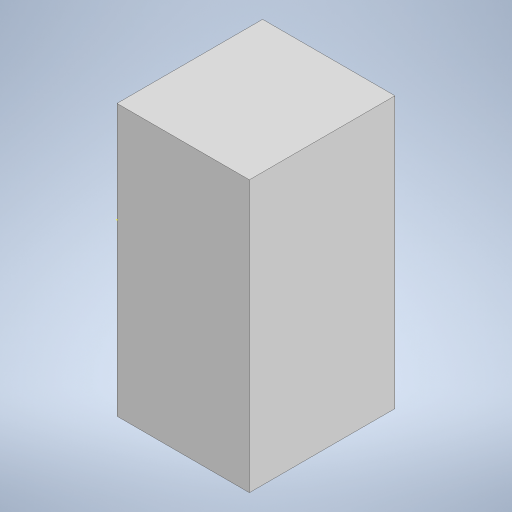
# Autodesk Inventor part: semaforoEsboço
Saved by Autodesk Inventor 2024 (Build 280153020, 153B)
## iProperties
Created: 2023-11-16
Part Number: semaforoEsboço
Material: Genérico
Document SubType Name: Modeling
Designer: a2625288
Density: 1 g/cm^3
Appearance: Padrão
Author: a2625288
Autodesk Inventor part; units mm, degrees
ref_plane "YZ Plane" through (0, 0, 0) normal (1, 0, 0) x (0, 1, 0)
ref_plane "XZ Plane" through (0, 0, 0) normal (0, 1, 0) x (-1, 0, 0)
ref_plane "XY Plane" through (0, 0, 0) normal (0, 0, 1) x (1, 0, 0)
sketch "Esboço1" plane through (0, 0, 0) normal (1, 0, 0) x (0, 1, 0)
  line L0 (10.9206, 18.8054) -> (-21.8794, 18.8054)
  line L1 (-21.8794, 18.8054) -> (-21.8794, 2.1054)
  line L2 (-21.8794, 2.1054) -> (10.9206, 2.1054)
  line L3 (10.9206, 2.1054) -> (10.9206, 18.8054)
  circle A0 centre (4.3506, 9.8054) radius 3.25
  circle A1 centre (4.3506, 9.8054) radius 3.8294
  circle A2 centre (-5.1194, 9.8054) radius 3.25
  circle A3 centre (-5.1194, 9.8054) radius 3.8763
  circle A4 centre (-14.5894, 9.8054) radius 3.25
  circle A5 centre (-14.5894, 9.8054) radius 3.9245
  point P0 (0, 0)
  point P1 (-5.4794, 18.8054)
  dimension "d0" = 32.8
  dimension "d1" = 16.7
  dimension "d2" = 32.8
  dimension "d7" = 6.5
  dimension "d8" = 6.5
  dimension "d9" = 6.5
  dimension "d22" = 9
  dimension "d23" = 9
  dimension "d24" = 9
  constraints: 8 end point, 6 centre point, 3 coincident, 2 perpendicular, 1 horizontal, 1 midpoint
  measures "d0" distance of L0.start L0.end
  measures "d1" distance of L0.end L1.end
  measures "d2" distance of L1.end L2.end
  measures "d7" diameter of A0
  measures "d8" diameter of A2
  measures "d9" diameter of A4
  measures "d22" distance from line of L0 A0.centre
  measures "d23" vertical distance of point (-5.479, 18.805) A2.centre
  measures "d24" distance from line of L0 A4.centre
extrude "Extrusão1" add sketch "Esboço1" along normal blind 3 contours L3 L2 L1 L0
sketch "Esboço2" plane through (0, -21.8794, 18.8054) normal (0, 0, 1) x (1, 0, 0)
  line L0 (3, 0) -> (3, 32.8) projected
  line L1 (0, 32.8) -> (3, 32.8) projected
  line L2 (3, 32.8) -> (15, 32.8)
  line L3 (15, 32.8) -> (15, 0)
  line L4 (15, 0) -> (3, 0)
  point P0 (0, 21.8794)
  dimension "d13" = 12
  constraints: 6 end point, 2 perpendicular, 1 horizontal
  measures "d13" distance of L0.end L2.end
extrude "Extrusão2" add sketch "Esboço2" against normal blind 2
sketch "Esboço3" plane through (0, -21.8794, 16.8054) normal (0, 0, -1) x (-1, 0, 0)
  line L0 (0, 32.8) -> (-3, 32.8) projected
  line L1 (0, 32.8) -> (-15, 32.8) projected
  line L2 (-3, 32.8) -> (-15, 32.8)
  line L3 (-15, 32.8) -> (-15, 0.0164)
  line L4 (-15, 0.0164) -> (-3, 0.0164)
  point P0 (0, 21.8794)
  constraints: 6 end point, 2 perpendicular, 1 collinear
sketch "Esboço4" plane through (0, -21.8794, 2.1054) normal (0, 0, -1) x (-1, 0, 0)
  line L0 (0, 32.8) -> (-3, 32.8) projected
  line L1 (0, 32.8) -> (-15, 32.8)
  line L2 (-15, 32.8) -> (-15, 0) projected
  line L3 (-15, 32.8) -> (-15, 0)
  line L4 (-15, 0) -> (0, 0)
  line L5 (0, 32.8) -> (0, 0) projected
  line L6 (0, 0) -> (0, 32.8)
  point P0 (0, 21.8794)
  constraints: 8 end point, 3 perpendicular, 1 collinear
extrude "Extrusão3" add sketch "Esboço4" along normal blind 2
sketch "Esboço5" plane through (0, 10.9206, 18.8054) normal (0, 1, 0) x (1, 0, 0)
  line L0 (0, 0) -> (15, 0) projected
  line L1 (15, 18.7) -> (0, 18.7) projected
  line L2 (15, 0) -> (15, 18.7)
  line L3 (15, 18.7) -> (0, 18.8054)
  line L4 (0, 18.8054) -> (0, 0)
  line L5 (0, 0) -> (15, 0)
  point P0 (0, 18.7)
  constraints: 8 end point, 1 parallel, 1 perpendicular, 1 vertical
extrude "Extrusão4" add sketch "Esboço5" along normal blind 2 contours L4 L1 L2 L0
sketch "Esboço6" plane through (15, -21.8794, 18.8054) normal (1, 0, 0) x (0, 0, -1)
  line L0 (0, 34.8) -> (18.7, 34.8) projected
  line L1 (0, 0) -> (0, 34.8) projected
  line L2 (0, 34.8) -> (0, 0)
  line L3 (0, 0) -> (18.7, 0)
  line L4 (18.7, 0) -> (18.7, 34.8) projected
  line L5 (18.7, 0) -> (18.7, 34.8)
  line L6 (18.7, 34.8) -> (0, 34.8)
  point P0 (18.8054, 21.8794)
  constraints: 8 end point, 3 perpendicular, 1 vertical
extrude "Extrusão5" add sketch "Esboço6" along normal blind 2
sketch "Esboço7" plane through (0, -21.8794, 18.8054) normal (0, 0, 1) x (1, 0, 0)
  point P0 (0, 21.8794)
